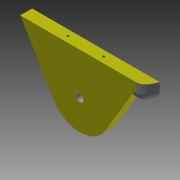
# Autodesk Inventor part: stojan2a
Saved by Autodesk Inventor 2015 (Build 190159000, 159)
## iProperties
Created: 2013-06-04
Part Number: stojan2a
Material: Generic
Document SubType Name: Modeling
Designer: idle-rug
Density: 1 g/cm^3
Appearance: Default
Author: idle-rug
Autodesk Inventor part; units mm, degrees
ref_plane "YZ Plane" through (0, 0, 0) normal (1, 0, 0) x (0, 1, 0)
ref_plane "XZ Plane" through (0, 0, 0) normal (0, 1, 0) x (-1, 0, 0)
ref_plane "XY Plane" through (0, 0, 0) normal (0, 0, 1) x (1, 0, 0)
sketch "Sketch1" plane through (0, 0, 0) normal (0, 1, 0) x (-1, 0, 0)
  circle A0 centre (0, -35) radius 25
  line L0 (0, 0) -> (50, 0)
  line L1 (50, 0) -> (-50, 0)
  line L2 (21.4679, -47.8113) -> (50, 0)
  line L3 (-21.4679, -47.8113) -> (-50, 0)
  circle A1 centre (0, -35) radius 3
  dimension "d4" = 50
  dimension "d5" = 50
  dimension "d6" = 100
  dimension "d7" = 6
  constraints: 8 end point, 2 centre point, 2 coincident, 2 point on circle, 2 tangent, 1 collinear, 1 horizontal, 1 point on line, 1 other
  measures "d4" diameter of A0
  measures "d5" distance of L0.start L0.end
  measures "d6" distance of L0.end L1.end
  measures "d7" diameter of A1
extrude "Extrusion1" add sketch "Sketch1" along normal blind 10
sketch "Sketch2" plane through (-50, 0, 0) normal (0, 0, 1) x (1, 0, 0)
  line L0 (0, 10) -> (100, 10) projected
  line L1 (0, 10) -> (50, 10)
  line L2 (50, 10) -> (50, 0)
  circle A0 centre (35, 5) radius 1
  circle A1 centre (65, 5) radius 1
  dimension "d11" = 2
  dimension "d12" = 2
  constraints: 4 end point, 2 centre point, 1 midpoint, 1 perpendicular
  measures "d11" diameter of A0
  measures "d12" diameter of A1
extrude "Extrusion2" cut sketch "Sketch2" against normal blind 10
sketch "Sketch3" plane through (0, 10, 0) normal (0, 1, 0) x (1, 0, 0)
  line L0 (51.0485, 0) -> (51.0485, 15)
  line L1 (51.0485, 15) -> (41.0485, 15)
  line L2 (50, 0) -> (21.4679, 47.8113) projected
  line L3 (41.0485, 15) -> (50, 0)
  line L4 (41.0485, 15) -> (50, 0)
  line L5 (50, 0) -> (51.0485, 0)
  point P0 (0, 0)
  dimension "d15" = 15
  dimension "d16" = 10
  constraints: 10 end point, 2 point on line, 1 collinear, 1 horizontal, 1 perpendicular, 1 vertical
  measures "d15" distance of L0.start L0.end
  measures "d16" distance of L0.end L1.end
extrude "Extrusion3" add sketch "Sketch3" against normal blind 10
sketch "Sketch4" plane through (51.0485, 10, 0) normal (1, 0, 0) x (0, 0, -1)
  line L0 (0, -10) -> (15, -10)
  line L1 (15, -10) -> (15, 0)
  line L2 (15, 0) -> (0, 0)
  line L3 (0, 0) -> (0, -10)
  constraints: 8 end point, 2 parallel, 1 horizontal, 1 perpendicular
extrude "Extrusion4" add sketch "Sketch4" along normal blind 6.4
sketch "Sketch5" plane through (-50, 0, 0) normal (0, 0, 1) x (1, 0, 0)
  line L0 (0, 10) -> (107.4485, 10) projected
  line L1 (50, 10) -> (50, 58.5)
  line L2 (50, 10) -> (98.5, 10) construction
  line L3 (0, 0) -> (107.4485, 0) projected
  line L4 (107.4485, 10) -> (91.0485, 10) projected
  arc A0 (101.6811, 0) -> (107.0608, 10) centre (50, 34.25) ccw
  line L5 (101.6811, 0) -> (107.4485, 0)
  line L6 (107.4485, 0) -> (107.4485, 10)
  line L7 (107.4485, 10) -> (107.4485, 0) projected
  arc A1 (101.6811, 0) -> (107.0608, 10) centre (50, 34.25) ccw
  line L8 (107.0608, 10) -> (107.4485, 10)
  line L9 (107.4485, 10) -> (107.4485, 0)
  arc A2 (101.6811, 0) -> (107.0608, 10) centre (50, 34.25) ccw
  point P0 (50, 0)
  dimension "d21" = 48.5
  dimension "d22" = 90
  constraints: 12 end point, 6 point on circle, 4 collinear, 3 centre point, 3 point on line, 2 perpendicular, 1 horizontal
  measures "d21" distance of L1.start L1.end
  measures "d22" angle of L2 L1
extrude "Extrusion5" cut sketch "Sketch5" against normal blind 15
fillet "Fillet1" radius 8 3 edges at (54.6004, 4.8766, -15) (51.6811, 0, -7.5) (46.3648, 0, -15)
body "Solid1"
